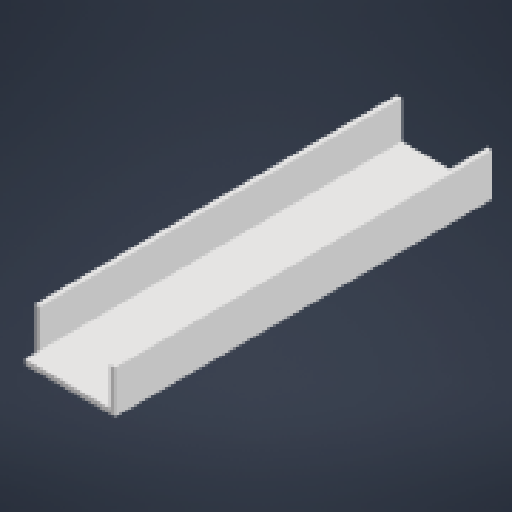
# Autodesk Inventor part: slide1
Saved by Autodesk Inventor 2026.2 (Build 302298000, 298)
## iProperties
Created: 2026-03-03
Part Number: slide1
Material: Generic
Document SubType Name: Modeling
Designer: shahd
Density: 1 g/cm^3
Appearance: Default
Author: shahd
Autodesk Inventor part; units mm, degrees
ref_plane "YZ Plane" through (0, 0, 0) normal (1, 0, 0) x (0, 1, 0)
ref_plane "XZ Plane" through (0, 0, 0) normal (0, 1, 0) x (-1, 0, 0)
ref_plane "XY Plane" through (0, 0, 0) normal (0, 0, 1) x (1, 0, 0)
sketch "Sketch1" plane through (0, 0, 0) normal (0, 0, 1) x (1, 0, 0)
  line L0 (0, 0) -> (-2, 0)
  line L1 (-2, 0) -> (36, 0)
  line L2 (36, 0) -> (36, 17)
  line L3 (36, 17) -> (34, 17)
  line L4 (34, 17) -> (34, 2)
  line L5 (34, 2) -> (0, 2)
  line L6 (0, 2) -> (0, 17)
  line L7 (0, 17) -> (-2, 17)
  line L8 (-2, 17) -> (-2, 0)
  dimension "d8" = 2
  dimension "d9" = 38
  dimension "d10" = 17
  dimension "d11" = 2
  dimension "d12" = 15
  constraints: 18 end point, 6 perpendicular, 3 point on line, 1 horizontal
  measures "d8" distance of L0.start L0.end
  measures "d9" distance of L0.end L1.end
  measures "d10" distance of L1.end L2.end
  measures "d11" distance of L2.end L3.end
  measures "d12" distance of L3.end L4.end
extrude "Extrusion1" add sketch "Sketch1" along normal blind 150
sketch "Sketch2" plane through (-2, 17, 150) normal (0, 1, 0) x (1, 0, 0)
  line L0 (0, 150) -> (0, 0) projected
  line L1 (0, 0) -> (0, 6)
  line L2 (0, 6) -> (2, 6)
  line L3 (2, 150) -> (2, 0) projected
  line L4 (2, 6) -> (2, 0)
  line L5 (2, 0) -> (0, 0)
  dimension "d13" = 6
  dimension "d14" = 2
  constraints: 8 end point, 2 point on line, 1 collinear, 1 perpendicular
  measures "d13" distance of L0.end L1.end
  measures "d14" distance of L1.end L2.end
extrude "Extrusion2" cut sketch "Sketch2" against normal through all
body "Solid1"
